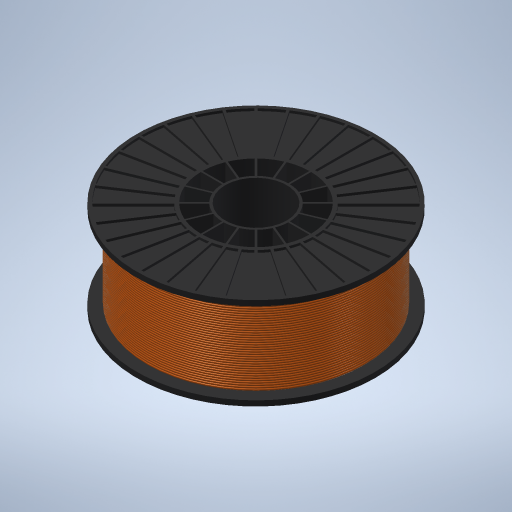
# Autodesk Inventor part: Sample Filament Spool
Saved by Autodesk Inventor 2024 (Build 280153000, 153)
## iProperties
Created: 2017-02-19
Part Number: Sample Filament Spool
Material: ABS Plastic
Document SubType Name: Modeling
Designer: Ishaan Govindarajan
Density: 1.06 g/cm^3
Appearance: Rubber - Black
Mass: 1663.72 g
Surface Area: 2295.81 cm^2
Volume: 1569.55 cm^3
Author: Ishaan Govindarajan
Autodesk Inventor part; units mm, degrees
ref_plane "YZ Plane" through (0, 0, 0) normal (1, 0, 0) x (0, 1, 0)
ref_plane "XZ Plane" through (0, 0, 0) normal (0, 1, 0) x (-1, 0, 0)
ref_plane "XY Plane" through (0, 0, 0) normal (0, 0, 1) x (1, 0, 0)
sketch "Sketch1" plane through (0, 0, 0) normal (0, 0, 1) x (1, 0, 0)
  circle A0 centre (0, 0) radius 101
  dimension "d0" = 202
  constraints: 1 centre point, 1 coincident
  measures "d0" diameter of A0
extrude "Extrusion1" add sketch "Sketch1" along normal mid plane 78
hole "Hole2" at (0, 0, 39) direction (0, 0, -1) diameter 52 end through all
sketch "Sketch4" plane through (0, 0, 39) normal (0, 0, 1) x (1, 0, 0)
  circle A0 centre (0, 0) radius 26 projected
  circle A1 centre (0, 0) radius 26 projected
  circle A2 centre (0, 0) radius 101 projected
  circle A3 centre (0, 0) radius 46
  circle A4 centre (0, 0) radius 28
  dimension "d22" = 20
  dimension "d23" = 2
  constraints: 2 centre point
  measures "d22" radial gap between concentric circles of A0 A3
  measures "d23" radial gap between concentric circles of A0 A4
extrude "Extrusion3" cut sketch "Sketch4" against normal blind 25 contours A3
sketch "Sketch5" plane through (0, 0, 39) normal (0, 0, 1) x (1, 0, 0)
  circle A0 centre (0, 0) radius 101 projected
  circle A1 centre (0, 0) radius 46 projected
  circle A2 centre (0, 0) radius 28 projected
  circle A3 centre (0, 0) radius 26 projected
  line L0 (-46, 0.75) -> (-27.99, 0.75)
  line L1 (-27.99, 0.75) -> (-27.99, -0.75)
  line L2 (-27.99, -0.75) -> (-46, -0.75)
  line L3 (-46, -0.75) -> (-46, 0.75)
  circle A4 centre (0, 0) radius 28 projected
  point P0 (-27.99, 0)
  dimension "d26" = 1.5
  constraints: 8 end point, 2 parallel, 1 horizontal, 1 horizontal alignment, 1 midpoint, 1 perpendicular, 1 tangent, 2 other
  measures "d26" distance of L2.end L0.start
extrude "Extrusion4" add sketch "Sketch5" against normal up to surface (25 mm away) contours L0 A2 L2 A1 | A1 L3 L0 | L2 L3 A1 | L1 A2 picked at (-33.9993, 0) picked at (-27.993, 0.0833)
pattern_circular "Circular Pattern1" count 16 over 360 about axis through (0, 0, -257.1284) along (0, 0, 1) of "Extrusion4"
sketch "Sketch6" plane through (0, 0, 39) normal (0, 0, 1) x (1, 0, 0)
  arc A0 (-33.0529, 31.9923) -> (-42.2058, 18.294) centre (0, 0) ccw projected
  line L0 (-20.3222, 19.2616) -> (-33.0529, 31.9923) projected
  arc A1 (-20.3222, 19.2616) -> (-25.5723, 11.4042) centre (0, 0) ccw projected
  line L1 (-42.2058, 18.294) -> (-25.5723, 11.4042) projected
  arc A2 (-18.294, 42.2058) -> (-31.9923, 33.0529) centre (0, 0) ccw projected
  line L2 (-11.4042, 25.5723) -> (-18.294, 42.2058) projected
  arc A3 (-11.4042, 25.5723) -> (-19.2616, 20.3222) centre (0, 0) ccw projected
  line L3 (-31.9923, 33.0529) -> (-19.2616, 20.3222) projected
  arc A4 (-0.75, 45.9939) -> (-16.9082, 42.7798) centre (0, 0) ccw projected
  line L4 (-0.75, 27.99) -> (-0.75, 45.9939) projected
  arc A5 (-0.75, 27.99) -> (-10.0184, 26.1464) centre (0, 0) ccw projected
  line L5 (-16.9082, 42.7798) -> (-10.0184, 26.1464) projected
  arc A6 (16.9082, 42.7798) -> (0.75, 45.9939) centre (0, 0) ccw projected
  line L6 (10.0184, 26.1464) -> (16.9082, 42.7798) projected
  arc A7 (10.0184, 26.1464) -> (0.75, 27.99) centre (0, 0) ccw projected
  line L7 (0.75, 45.9939) -> (0.75, 27.99) projected
  arc A8 (31.9923, 33.0529) -> (18.294, 42.2058) centre (0, 0) ccw projected
  line L8 (19.2616, 20.3222) -> (31.9923, 33.0529) projected
  arc A9 (19.2616, 20.3222) -> (11.4042, 25.5723) centre (0, 0) ccw projected
  line L9 (18.294, 42.2058) -> (11.4042, 25.5723) projected
  arc A10 (42.2058, 18.294) -> (33.0529, 31.9923) centre (0, 0) ccw projected
  line L10 (25.5723, 11.4042) -> (42.2058, 18.294) projected
  arc A11 (25.5723, 11.4042) -> (20.3222, 19.2616) centre (0, 0) ccw projected
  line L11 (33.0529, 31.9923) -> (20.3222, 19.2616) projected
  arc A12 (45.9939, 0.75) -> (42.7798, 16.9082) centre (0, 0) ccw projected
  line L12 (27.99, 0.75) -> (45.9939, 0.75) projected
  arc A13 (27.99, 0.75) -> (26.1464, 10.0184) centre (0, 0) ccw projected
  line L13 (42.7798, 16.9082) -> (26.1464, 10.0184) projected
  arc A14 (42.7798, -16.9082) -> (45.9939, -0.75) centre (0, 0) ccw projected
  line L14 (26.1464, -10.0184) -> (42.7798, -16.9082) projected
  arc A15 (26.1464, -10.0184) -> (27.99, -0.75) centre (0, 0) ccw projected
  line L15 (45.9939, -0.75) -> (27.99, -0.75) projected
  arc A16 (33.0529, -31.9923) -> (42.2058, -18.294) centre (0, 0) ccw projected
  line L16 (20.3222, -19.2616) -> (33.0529, -31.9923) projected
  arc A17 (20.3222, -19.2616) -> (25.5723, -11.4042) centre (0, 0) ccw projected
  line L17 (42.2058, -18.294) -> (25.5723, -11.4042) projected
  arc A18 (18.294, -42.2058) -> (31.9923, -33.0529) centre (0, 0) ccw projected
  line L18 (11.4042, -25.5723) -> (18.294, -42.2058) projected
  arc A19 (11.4042, -25.5723) -> (19.2616, -20.3222) centre (0, 0) ccw projected
  line L19 (31.9923, -33.0529) -> (19.2616, -20.3222) projected
  arc A20 (0.75, -45.9939) -> (16.9082, -42.7798) centre (0, 0) ccw projected
  line L20 (0.75, -27.99) -> (0.75, -45.9939) projected
  arc A21 (0.75, -27.99) -> (10.0184, -26.1464) centre (0, 0) ccw projected
  line L21 (16.9082, -42.7798) -> (10.0184, -26.1464) projected
  arc A22 (-16.9082, -42.7798) -> (-0.75, -45.9939) centre (0, 0) ccw projected
  line L22 (-10.0184, -26.1464) -> (-16.9082, -42.7798) projected
  arc A23 (-10.0184, -26.1464) -> (-0.75, -27.99) centre (0, 0) ccw projected
  line L23 (-0.75, -45.9939) -> (-0.75, -27.99) projected
  arc A24 (-31.9923, -33.0529) -> (-18.294, -42.2058) centre (0, 0) ccw projected
  line L24 (-19.2616, -20.3222) -> (-31.9923, -33.0529) projected
  arc A25 (-19.2616, -20.3222) -> (-11.4042, -25.5723) centre (0, 0) ccw projected
  line L25 (-18.294, -42.2058) -> (-11.4042, -25.5723) projected
  arc A26 (-42.2058, -18.294) -> (-33.0529, -31.9923) centre (0, 0) ccw projected
  line L26 (-25.5723, -11.4042) -> (-42.2058, -18.294) projected
  arc A27 (-25.5723, -11.4042) -> (-20.3222, -19.2616) centre (0, 0) ccw projected
  line L27 (-33.0529, -31.9923) -> (-20.3222, -19.2616) projected
  arc A28 (-45.9939, -0.75) -> (-42.7798, -16.9082) centre (0, 0) ccw projected
  line L28 (-27.99, -0.75) -> (-45.9939, -0.75) projected
  arc A29 (-27.99, -0.75) -> (-26.1464, -10.0184) centre (0, 0) ccw projected
  line L29 (-42.7798, -16.9082) -> (-26.1464, -10.0184) projected
  line L30 (-26.1464, 10.0184) -> (-42.7798, 16.9082) projected
  arc A30 (-26.1464, 10.0184) -> (-27.99, 0.75) centre (0, 0) ccw projected
  line L31 (-45.9939, 0.75) -> (-27.99, 0.75) projected
  arc A31 (-42.7798, 16.9082) -> (-45.9939, 0.75) centre (0, 0) ccw projected
  circle A32 centre (0, 0) radius 101 projected
  circle A33 centre (0, 0) radius 26 projected
  circle A34 centre (0, 0) radius 49
  circle A35 centre (0, 0) radius 98
  dimension "d32" = 3
  dimension "d33" = 3
  constraints: 2 centre point
  measures "d32" radial gap between concentric circles of A6 A34
  measures "d33" radial gap between concentric circles of A32 A35
extrude "Extrusion5" cut sketch "Sketch6" against normal blind 2 contours A35
sketch "Sketch7" plane through (0, 0, 37) normal (0, 0, 1) x (1, 0, 0)
  circle A0 centre (0, 0) radius 49 projected
  circle A1 centre (0, 0) radius 98 projected
  line L0 (-48.9898, 1) -> (-98, 1)
  line L1 (-98, 1) -> (-98, -1)
  line L2 (-98, -1) -> (-48.9898, -1)
  line L3 (-48.9898, -1) -> (-48.9898, 1)
  dimension "d36" = 2
  constraints: 8 end point, 2 parallel, 2 point on circle, 1 horizontal, 1 perpendicular, 1 tangent
  measures "d36" distance between parallel lines of L2 L0
extrude "Extrusion6" add sketch "Sketch7" along normal up to surface (2 mm away) contours A0 L2 A1 L0 | A1 L1 L0 | L2 L1 A1 picked at (-65.3326, 0)
pattern_circular "Circular Pattern2" count 32 over 360 about axis through (0, 0, 39) along (0, 0, -1) of "Extrusion6"
mirror "Mirror1" about plane through (0, 0, 0) normal (0, 0, 1) of "Extrusion3", "Extrusion4", "Circular Pattern1", "Extrusion5", "Extrusion6", "Circular Pattern2"
sketch "Sketch8" plane through (0, 0, -39) normal (0, 0, -1) x (-1, 0, 0)
  arc A0 (90.9182, -36.5771) -> (95.9169, -20.0986) centre (0, 0) ccw projected
  line L0 (90.9182, -36.5771) -> (45.6434, -17.8237) projected
  arc A1 (45.6434, -17.8237) -> (47.8534, -10.5382) centre (0, 0) ccw projected
  line L1 (47.8534, -10.5382) -> (95.9169, -20.0986) projected
  arc A2 (82.0353, -53.6116) -> (90.1528, -38.4249) centre (0, 0) ccw projected
  line L2 (82.0353, -53.6116) -> (41.2891, -26.3858) projected
  arc A3 (41.2891, -26.3858) -> (44.878, -19.6715) centre (0, 0) ccw projected
  line L3 (44.878, -19.6715) -> (90.1528, -38.4249) projected
  arc A4 (70, -68.5857) -> (80.9242, -55.2745) centre (0, 0) ccw projected
  line L4 (70, -68.5857) -> (35.3481, -33.9339) projected
  arc A5 (35.3481, -33.9339) -> (40.178, -28.0487) centre (0, 0) ccw projected
  line L5 (40.178, -28.0487) -> (80.9242, -55.2745) projected
  arc A6 (55.2745, -80.9242) -> (68.5857, -70) centre (0, 0) ccw projected
  line L6 (55.2745, -80.9242) -> (28.0487, -40.178) projected
  arc A7 (28.0487, -40.178) -> (33.9339, -35.3481) centre (0, 0) ccw projected
  line L7 (33.9339, -35.3481) -> (68.5857, -70) projected
  arc A8 (38.4249, -90.1528) -> (53.6116, -82.0353) centre (0, 0) ccw projected
  line L8 (38.4249, -90.1528) -> (19.6715, -44.878) projected
  arc A9 (19.6715, -44.878) -> (26.3858, -41.2891) centre (0, 0) ccw projected
  line L9 (26.3858, -41.2891) -> (53.6116, -82.0353) projected
  arc A10 (20.0986, -95.9169) -> (36.5771, -90.9182) centre (0, 0) ccw projected
  line L10 (20.0986, -95.9169) -> (10.5382, -47.8534) projected
  arc A11 (10.5382, -47.8534) -> (17.8237, -45.6434) centre (0, 0) ccw projected
  line L11 (17.8237, -45.6434) -> (36.5771, -90.9182) projected
  arc A12 (1, -97.9949) -> (18.1371, -96.307) centre (0, 0) ccw projected
  line L12 (1, -97.9949) -> (1, -48.9898) projected
  arc A13 (1, -48.9898) -> (8.5766, -48.2436) centre (0, 0) ccw projected
  line L13 (8.5766, -48.2436) -> (18.1371, -96.307) projected
  arc A14 (-18.1371, -96.307) -> (-1, -97.9949) centre (0, 0) ccw projected
  line L14 (-18.1371, -96.307) -> (-8.5766, -48.2436) projected
  arc A15 (-8.5766, -48.2436) -> (-1, -48.9898) centre (0, 0) ccw projected
  line L15 (-1, -48.9898) -> (-1, -97.9949) projected
  arc A16 (-36.5771, -90.9182) -> (-20.0986, -95.9169) centre (0, 0) ccw projected
  line L16 (-36.5771, -90.9182) -> (-17.8237, -45.6434) projected
  arc A17 (-17.8237, -45.6434) -> (-10.5382, -47.8534) centre (0, 0) ccw projected
  line L17 (-10.5382, -47.8534) -> (-20.0986, -95.9169) projected
  arc A18 (-53.6116, -82.0353) -> (-38.4249, -90.1528) centre (0, 0) ccw projected
  line L18 (-53.6116, -82.0353) -> (-26.3858, -41.2891) projected
  arc A19 (-26.3858, -41.2891) -> (-19.6715, -44.878) centre (0, 0) ccw projected
  line L19 (-19.6715, -44.878) -> (-38.4249, -90.1528) projected
  arc A20 (-68.5857, -70) -> (-55.2745, -80.9242) centre (0, 0) ccw projected
  line L20 (-68.5857, -70) -> (-33.9339, -35.3481) projected
  arc A21 (-33.9339, -35.3481) -> (-28.0487, -40.178) centre (0, 0) ccw projected
  line L21 (-28.0487, -40.178) -> (-55.2745, -80.9242) projected
  arc A22 (-80.9242, -55.2745) -> (-70, -68.5857) centre (0, 0) ccw projected
  line L22 (-80.9242, -55.2745) -> (-40.178, -28.0487) projected
  arc A23 (-40.178, -28.0487) -> (-35.3481, -33.9339) centre (0, 0) ccw projected
  line L23 (-35.3481, -33.9339) -> (-70, -68.5857) projected
  arc A24 (-90.1528, -38.4249) -> (-82.0353, -53.6116) centre (0, 0) ccw projected
  line L24 (-90.1528, -38.4249) -> (-44.878, -19.6715) projected
  arc A25 (-44.878, -19.6715) -> (-41.2891, -26.3858) centre (0, 0) ccw projected
  line L25 (-41.2891, -26.3858) -> (-82.0353, -53.6116) projected
  arc A26 (-95.9169, -20.0986) -> (-90.9182, -36.5771) centre (0, 0) ccw projected
  line L26 (-95.9169, -20.0986) -> (-47.8534, -10.5382) projected
  arc A27 (-47.8534, -10.5382) -> (-45.6434, -17.8237) centre (0, 0) ccw projected
  line L27 (-45.6434, -17.8237) -> (-90.9182, -36.5771) projected
  arc A28 (-97.9949, -1) -> (-96.307, -18.1371) centre (0, 0) ccw projected
  line L28 (-97.9949, -1) -> (-48.9898, -1) projected
  arc A29 (-48.9898, -1) -> (-48.2436, -8.5766) centre (0, 0) ccw projected
  line L29 (-48.2436, -8.5766) -> (-96.307, -18.1371) projected
  arc A30 (-96.307, 18.1371) -> (-97.9949, 1) centre (0, 0) ccw projected
  line L30 (-96.307, 18.1371) -> (-48.2436, 8.5766) projected
  arc A31 (-48.2436, 8.5766) -> (-48.9898, 1) centre (0, 0) ccw projected
  line L31 (-48.9898, 1) -> (-97.9949, 1) projected
  arc A32 (-90.9182, 36.5771) -> (-95.9169, 20.0986) centre (0, 0) ccw projected
  line L32 (-90.9182, 36.5771) -> (-45.6434, 17.8237) projected
  arc A33 (-45.6434, 17.8237) -> (-47.8534, 10.5382) centre (0, 0) ccw projected
  line L33 (-47.8534, 10.5382) -> (-95.9169, 20.0986) projected
  arc A34 (-82.0353, 53.6116) -> (-90.1528, 38.4249) centre (0, 0) ccw projected
  line L34 (-82.0353, 53.6116) -> (-41.2891, 26.3858) projected
  arc A35 (-41.2891, 26.3858) -> (-44.878, 19.6715) centre (0, 0) ccw projected
  line L35 (-44.878, 19.6715) -> (-90.1528, 38.4249) projected
  arc A36 (-70, 68.5857) -> (-80.9242, 55.2745) centre (0, 0) ccw projected
  line L36 (-70, 68.5857) -> (-35.3481, 33.9339) projected
  arc A37 (-35.3481, 33.9339) -> (-40.178, 28.0487) centre (0, 0) ccw projected
  line L37 (-40.178, 28.0487) -> (-80.9242, 55.2745) projected
  arc A38 (-55.2745, 80.9242) -> (-68.5857, 70) centre (0, 0) ccw projected
  line L38 (-55.2745, 80.9242) -> (-28.0487, 40.178) projected
  arc A39 (-28.0487, 40.178) -> (-33.9339, 35.3481) centre (0, 0) ccw projected
  line L39 (-33.9339, 35.3481) -> (-68.5857, 70) projected
  arc A40 (-38.4249, 90.1528) -> (-53.6116, 82.0353) centre (0, 0) ccw projected
  line L40 (-38.4249, 90.1528) -> (-19.6715, 44.878) projected
  arc A41 (-19.6715, 44.878) -> (-26.3858, 41.2891) centre (0, 0) ccw projected
  line L41 (-26.3858, 41.2891) -> (-53.6116, 82.0353) projected
  arc A42 (-20.0986, 95.9169) -> (-36.5771, 90.9182) centre (0, 0) ccw projected
  line L42 (-20.0986, 95.9169) -> (-10.5382, 47.8534) projected
  arc A43 (-10.5382, 47.8534) -> (-17.8237, 45.6434) centre (0, 0) ccw projected
  line L43 (-17.8237, 45.6434) -> (-36.5771, 90.9182) projected
  arc A44 (-1, 97.9949) -> (-18.1371, 96.307) centre (0, 0) ccw projected
  line L44 (-1, 97.9949) -> (-1, 48.9898) projected
  arc A45 (-1, 48.9898) -> (-8.5766, 48.2436) centre (0, 0) ccw projected
  line L45 (-8.5766, 48.2436) -> (-18.1371, 96.307) projected
  arc A46 (18.1371, 96.307) -> (1, 97.9949) centre (0, 0) ccw projected
  line L46 (18.1371, 96.307) -> (8.5766, 48.2436) projected
  arc A47 (8.5766, 48.2436) -> (1, 48.9898) centre (0, 0) ccw projected
  line L47 (1, 48.9898) -> (1, 97.9949) projected
  arc A48 (36.5771, 90.9182) -> (20.0986, 95.9169) centre (0, 0) ccw projected
  line L48 (36.5771, 90.9182) -> (17.8237, 45.6434) projected
  arc A49 (17.8237, 45.6434) -> (10.5382, 47.8534) centre (0, 0) ccw projected
  line L49 (10.5382, 47.8534) -> (20.0986, 95.9169) projected
  arc A50 (53.6116, 82.0353) -> (38.4249, 90.1528) centre (0, 0) ccw projected
  line L50 (53.6116, 82.0353) -> (26.3858, 41.2891) projected
  arc A51 (26.3858, 41.2891) -> (19.6715, 44.878) centre (0, 0) ccw projected
  line L51 (19.6715, 44.878) -> (38.4249, 90.1528) projected
  arc A52 (68.5857, 70) -> (55.2745, 80.9242) centre (0, 0) ccw projected
  line L52 (68.5857, 70) -> (33.9339, 35.3481) projected
  arc A53 (33.9339, 35.3481) -> (28.0487, 40.178) centre (0, 0) ccw projected
  line L53 (28.0487, 40.178) -> (55.2745, 80.9242) projected
  arc A54 (80.9242, 55.2745) -> (70, 68.5857) centre (0, 0) ccw projected
  line L54 (80.9242, 55.2745) -> (40.178, 28.0487) projected
  arc A55 (40.178, 28.0487) -> (35.3481, 33.9339) centre (0, 0) ccw projected
  line L55 (35.3481, 33.9339) -> (70, 68.5857) projected
  arc A56 (90.1528, 38.4249) -> (82.0353, 53.6116) centre (0, 0) ccw projected
  line L56 (90.1528, 38.4249) -> (44.878, 19.6715) projected
  arc A57 (44.878, 19.6715) -> (41.2891, 26.3858) centre (0, 0) ccw projected
  line L57 (41.2891, 26.3858) -> (82.0353, 53.6116) projected
  arc A58 (95.9169, 20.0986) -> (90.9182, 36.5771) centre (0, 0) ccw projected
  line L58 (95.9169, 20.0986) -> (47.8534, 10.5382) projected
  arc A59 (47.8534, 10.5382) -> (45.6434, 17.8237) centre (0, 0) ccw projected
  line L59 (45.6434, 17.8237) -> (90.9182, 36.5771) projected
  arc A60 (97.9949, 1) -> (96.307, 18.1371) centre (0, 0) ccw projected
  line L60 (97.9949, 1) -> (48.9898, 1) projected
  arc A61 (48.9898, 1) -> (48.2436, 8.5766) centre (0, 0) ccw projected
  line L61 (48.2436, 8.5766) -> (96.307, 18.1371) projected
  line L62 (42.7798, -16.9082) -> (26.1464, -10.0184) projected
  arc A62 (26.1464, -10.0184) -> (27.99, -0.75) centre (0, 0) ccw projected
  line L63 (27.99, -0.75) -> (45.9939, -0.75) projected
  arc A63 (42.7798, -16.9082) -> (45.9939, -0.75) centre (0, 0) ccw projected
  circle A64 centre (0, 0) radius 26 projected
  line L64 (33.0529, -31.9923) -> (20.3222, -19.2616) projected
  arc A65 (20.3222, -19.2616) -> (25.5723, -11.4042) centre (0, 0) ccw projected
  line L65 (25.5723, -11.4042) -> (42.2058, -18.294) projected
  arc A66 (33.0529, -31.9923) -> (42.2058, -18.294) centre (0, 0) ccw projected
  line L66 (18.294, -42.2058) -> (11.4042, -25.5723) projected
  arc A67 (11.4042, -25.5723) -> (19.2616, -20.3222) centre (0, 0) ccw projected
  line L67 (19.2616, -20.3222) -> (31.9923, -33.0529) projected
  arc A68 (18.294, -42.2058) -> (31.9923, -33.0529) centre (0, 0) ccw projected
  line L68 (0.75, -45.9939) -> (0.75, -27.99) projected
  arc A69 (0.75, -27.99) -> (10.0184, -26.1464) centre (0, 0) ccw projected
  line L69 (10.0184, -26.1464) -> (16.9082, -42.7798) projected
  arc A70 (0.75, -45.9939) -> (16.9082, -42.7798) centre (0, 0) ccw projected
  line L70 (-16.9082, -42.7798) -> (-10.0184, -26.1464) projected
  arc A71 (-10.0184, -26.1464) -> (-0.75, -27.99) centre (0, 0) ccw projected
  line L71 (-0.75, -27.99) -> (-0.75, -45.9939) projected
  arc A72 (-16.9082, -42.7798) -> (-0.75, -45.9939) centre (0, 0) ccw projected
  line L72 (-31.9923, -33.0529) -> (-19.2616, -20.3222) projected
  arc A73 (-19.2616, -20.3222) -> (-11.4042, -25.5723) centre (0, 0) ccw projected
  line L73 (-11.4042, -25.5723) -> (-18.294, -42.2058) projected
  arc A74 (-31.9923, -33.0529) -> (-18.294, -42.2058) centre (0, 0) ccw projected
  line L74 (-42.2058, -18.294) -> (-25.5723, -11.4042) projected
  arc A75 (-25.5723, -11.4042) -> (-20.3222, -19.2616) centre (0, 0) ccw projected
  line L75 (-20.3222, -19.2616) -> (-33.0529, -31.9923) projected
  arc A76 (-42.2058, -18.294) -> (-33.0529, -31.9923) centre (0, 0) ccw projected
  line L76 (-45.9939, -0.75) -> (-27.99, -0.75) projected
  arc A77 (-27.99, -0.75) -> (-26.1464, -10.0184) centre (0, 0) ccw projected
  line L77 (-26.1464, -10.0184) -> (-42.7798, -16.9082) projected
  arc A78 (-45.9939, -0.75) -> (-42.7798, -16.9082) centre (0, 0) ccw projected
  line L78 (-42.7798, 16.9082) -> (-26.1464, 10.0184) projected
  arc A79 (-26.1464, 10.0184) -> (-27.99, 0.75) centre (0, 0) ccw projected
  line L79 (-27.99, 0.75) -> (-45.9939, 0.75) projected
  arc A80 (-42.7798, 16.9082) -> (-45.9939, 0.75) centre (0, 0) ccw projected
  line L80 (-33.0529, 31.9923) -> (-20.3222, 19.2616) projected
  arc A81 (-20.3222, 19.2616) -> (-25.5723, 11.4042) centre (0, 0) ccw projected
  line L81 (-25.5723, 11.4042) -> (-42.2058, 18.294) projected
  arc A82 (-33.0529, 31.9923) -> (-42.2058, 18.294) centre (0, 0) ccw projected
  line L82 (-18.294, 42.2058) -> (-11.4042, 25.5723) projected
  arc A83 (-11.4042, 25.5723) -> (-19.2616, 20.3222) centre (0, 0) ccw projected
  line L83 (-19.2616, 20.3222) -> (-31.9923, 33.0529) projected
  arc A84 (-18.294, 42.2058) -> (-31.9923, 33.0529) centre (0, 0) ccw projected
  line L84 (-0.75, 45.9939) -> (-0.75, 27.99) projected
  arc A85 (-0.75, 27.99) -> (-10.0184, 26.1464) centre (0, 0) ccw projected
  line L85 (-10.0184, 26.1464) -> (-16.9082, 42.7798) projected
  arc A86 (-0.75, 45.9939) -> (-16.9082, 42.7798) centre (0, 0) ccw projected
  line L86 (16.9082, 42.7798) -> (10.0184, 26.1464) projected
  arc A87 (10.0184, 26.1464) -> (0.75, 27.99) centre (0, 0) ccw projected
  line L87 (0.75, 27.99) -> (0.75, 45.9939) projected
  arc A88 (16.9082, 42.7798) -> (0.75, 45.9939) centre (0, 0) ccw projected
  line L88 (31.9923, 33.0529) -> (19.2616, 20.3222) projected
  arc A89 (19.2616, 20.3222) -> (11.4042, 25.5723) centre (0, 0) ccw projected
  line L89 (11.4042, 25.5723) -> (18.294, 42.2058) projected
  arc A90 (31.9923, 33.0529) -> (18.294, 42.2058) centre (0, 0) ccw projected
  line L90 (42.2058, 18.294) -> (25.5723, 11.4042) projected
  arc A91 (25.5723, 11.4042) -> (20.3222, 19.2616) centre (0, 0) ccw projected
  line L91 (20.3222, 19.2616) -> (33.0529, 31.9923) projected
  arc A92 (42.2058, 18.294) -> (33.0529, 31.9923) centre (0, 0) ccw projected
  arc A93 (45.9939, 0.75) -> (42.7798, 16.9082) centre (0, 0) ccw projected
  line L92 (45.9939, 0.75) -> (27.99, 0.75) projected
  arc A94 (27.99, 0.75) -> (26.1464, 10.0184) centre (0, 0) ccw projected
  line L93 (26.1464, 10.0184) -> (42.7798, 16.9082) projected
  line L94 (96.307, -18.1371) -> (48.2436, -8.5766) projected
  arc A95 (48.2436, -8.5766) -> (48.9898, -1) centre (0, 0) ccw projected
  line L95 (48.9898, -1) -> (97.9949, -1) projected
  arc A96 (96.307, -18.1371) -> (97.9949, -1) centre (0, 0) ccw projected
  circle A97 centre (0, 0) radius 101 projected
  circle A98 centre (0, 0) radius 46
  constraints: 1 coincident, 3 other
extrude "Extrusion7" cut sketch "Sketch8" against normal blind 16 contours A98 L65 A65 L64 L67 A67 L66 L69 A69 L68 L71 A71 L70 L73 A73 L72 L75 A75 L74 L77 A77 L76 L79 A79 L78 L81 A81 L80 L83 A83 L82 L85 A85 L84 L87 A87 L86 L89 A89 L88 L91 A91 L90 L93 A94 L92 L63 A62 L62
sketch "Sketch9" plane through (42.2058, -18.294, -14) normal (0, 0, -1) x (-0.9238795, 0.3826834, 0)
  line L0 (14.0016, 33.8029) -> (26.7323, 21.0722) projected
  arc A0 (34.5897, 26.3223) -> (26.7323, 21.0722) centre (45.9939, 0.75) ccw projected
  line L1 (34.5897, 26.3223) -> (27.6999, 42.9558) projected
  arc A1 (27.6999, 42.9558) -> (14.0016, 33.8029) centre (45.9939, 0.75) ccw projected
  line L2 (29.0857, 43.5298) -> (35.9755, 26.8964) projected
  arc A2 (45.2439, 28.74) -> (35.9755, 26.8964) centre (45.9939, 0.75) ccw projected
  line L3 (45.2439, 28.74) -> (45.2439, 46.7439) projected
  arc A3 (45.2439, 46.7439) -> (29.0857, 43.5298) centre (45.9939, 0.75) ccw projected
  line L4 (46.7439, 46.7439) -> (46.7439, 28.74) projected
  arc A4 (56.0123, 26.8964) -> (46.7439, 28.74) centre (45.9939, 0.75) ccw projected
  line L5 (56.0123, 26.8964) -> (62.9021, 43.5298) projected
  arc A5 (62.9021, 43.5298) -> (46.7439, 46.7439) centre (45.9939, 0.75) ccw projected
  line L6 (64.2879, 42.9558) -> (57.3981, 26.3223) projected
  arc A6 (65.2554, 21.0722) -> (57.3981, 26.3223) centre (45.9939, 0.75) ccw projected
  line L7 (65.2554, 21.0722) -> (77.9861, 33.8029) projected
  arc A7 (77.9861, 33.8029) -> (64.2879, 42.9558) centre (45.9939, 0.75) ccw projected
  line L8 (79.0468, 32.7423) -> (66.3161, 20.0116) projected
  arc A8 (71.5662, 12.1542) -> (66.3161, 20.0116) centre (45.9939, 0.75) ccw projected
  line L9 (71.5662, 12.1542) -> (88.1997, 19.044) projected
  arc A9 (88.1997, 19.044) -> (79.0468, 32.7423) centre (45.9939, 0.75) ccw projected
  line L10 (88.7737, 17.6582) -> (72.1402, 10.7684) projected
  arc A10 (73.9838, 1.5) -> (72.1402, 10.7684) centre (45.9939, 0.75) ccw projected
  line L11 (73.9838, 1.5) -> (91.9878, 1.5) projected
  arc A11 (91.9878, 1.5) -> (88.7737, 17.6582) centre (45.9939, 0.75) ccw projected
  line L12 (91.9878, 0) -> (73.9838, 0) projected
  arc A12 (72.1402, -9.2684) -> (73.9838, 0) centre (45.9939, 0.75) ccw projected
  line L13 (72.1402, -9.2684) -> (88.7737, -16.1582) projected
  arc A13 (88.7737, -16.1582) -> (91.9878, 0) centre (45.9939, 0.75) ccw projected
  line L14 (88.1997, -17.544) -> (71.5662, -10.6542) projected
  arc A14 (66.3161, -18.5116) -> (71.5662, -10.6542) centre (45.9939, 0.75) ccw projected
  line L15 (66.3161, -18.5116) -> (79.0468, -31.2423) projected
  arc A15 (79.0468, -31.2423) -> (88.1997, -17.544) centre (45.9939, 0.75) ccw projected
  line L16 (3.7881, 19.044) -> (20.4216, 12.1542) projected
  arc A16 (25.6717, 20.0116) -> (20.4216, 12.1542) centre (45.9939, 0.75) ccw projected
  line L17 (25.6717, 20.0116) -> (12.941, 32.7423) projected
  arc A17 (12.941, 32.7423) -> (3.7881, 19.044) centre (45.9939, 0.75) ccw projected
  line L18 (0, 1.5) -> (18.0039, 1.5) projected
  arc A18 (19.8475, 10.7684) -> (18.0039, 1.5) centre (45.9939, 0.75) ccw projected
  line L19 (19.8475, 10.7684) -> (3.2141, 17.6582) projected
  arc A19 (3.2141, 17.6582) -> (0, 1.5) centre (45.9939, 0.75) ccw projected
  line L20 (3.2141, -16.1582) -> (19.8475, -9.2684) projected
  arc A20 (18.0039, 0) -> (19.8475, -9.2684) centre (45.9939, 0.75) ccw projected
  line L21 (18.0039, 0) -> (0, 0) projected
  arc A21 (0, 0) -> (3.2141, -16.1582) centre (45.9939, 0.75) ccw projected
  line L22 (12.941, -31.2423) -> (25.6717, -18.5116) projected
  arc A22 (20.4216, -10.6542) -> (25.6717, -18.5116) centre (45.9939, 0.75) ccw projected
  line L23 (20.4216, -10.6542) -> (3.7881, -17.544) projected
  arc A23 (3.7881, -17.544) -> (12.941, -31.2423) centre (45.9939, 0.75) ccw projected
  line L24 (27.6999, -41.4558) -> (34.5897, -24.8223) projected
  arc A24 (26.7323, -19.5722) -> (34.5897, -24.8223) centre (45.9939, 0.75) ccw projected
  line L25 (26.7323, -19.5722) -> (14.0016, -32.3029) projected
  arc A25 (14.0016, -32.3029) -> (27.6999, -41.4558) centre (45.9939, 0.75) ccw projected
  line L26 (45.2439, -45.2439) -> (45.2439, -27.24) projected
  arc A26 (35.9755, -25.3964) -> (45.2439, -27.24) centre (45.9939, 0.75) ccw projected
  line L27 (35.9755, -25.3964) -> (29.0857, -42.0298) projected
  arc A27 (29.0857, -42.0298) -> (45.2439, -45.2439) centre (45.9939, 0.75) ccw projected
  line L28 (57.3981, -24.8223) -> (64.2879, -41.4558) projected
  arc A28 (64.2879, -41.4558) -> (77.9861, -32.3029) centre (45.9939, 0.75) ccw projected
  line L29 (77.9861, -32.3029) -> (65.2554, -19.5722) projected
  arc A29 (57.3981, -24.8223) -> (65.2554, -19.5722) centre (45.9939, 0.75) ccw projected
  line L30 (62.9021, -42.0298) -> (56.0123, -25.3964) projected
  arc A30 (46.7439, -27.24) -> (56.0123, -25.3964) centre (45.9939, 0.75) ccw projected
  line L31 (46.7439, -27.24) -> (46.7439, -45.2439) projected
  arc A31 (46.7439, -45.2439) -> (62.9021, -42.0298) centre (45.9939, 0.75) ccw projected
  circle A32 centre (45.9939, 0.75) radius 26 projected
  circle A33 centre (45.9939, 0.75) radius 101 projected
extrude "Extrusion8" cut sketch "Sketch9" against normal blind 26 contours A1 L1 A0 L0 | A3 L3 A2 L2 | A5 L5 A4 L4 | A7 L7 A6 L6 | A9 L9 A8 L8 | A11 L11 A10 L10 | A13 L13 A12 L12 | A15 L15 A14 L14 | A17 L17 A16 L16 | A19 L19 A18 L18 | A21 L21 A20 L20 | A23 L23 A22 L22 | A25 L25 A24 L24 | A27 L27 A26 L26 | A29 L29 A28 L28 | A31 L31 A30 L30
sketch "Sketch10" plane through (0, 0, 0) normal (1, 0, 0) x (0, 1, 0)
  line L0 (-101, 39) -> (-26, 39) projected
  line L1 (-26, 39) -> (-26, -23) projected
  line L2 (-26, -23) -> (-46, -23) projected
  line L3 (-46, -23) -> (-46, -39) projected
  line L4 (-46, -39) -> (-101, -39) projected
  line L5 (-101, -39) -> (-101, 39) projected
  line L6 (26, 39) -> (101, 39) projected
  line L7 (101, 39) -> (101, -39) projected
  line L8 (101, -39) -> (46, -39) projected
  line L9 (46, -39) -> (46, -23) projected
  line L10 (46, -23) -> (26, -23) projected
  line L11 (26, -23) -> (26, 39) projected
  line L12 (101, -34.5) -> (91, -34.5)
  line L13 (91, -34.5) -> (91, 34.5)
  line L14 (91, 34.5) -> (101, 34.5)
  line L15 (101, 34.5) -> (101, -34.5)
  line L16 (0, -54.6) -> (0, 54.6) projected
  point P0 (0, 0)
  dimension "d46" = 4.5
  dimension "d47" = 4.5
  dimension "d48" = 10
  constraints: 8 end point, 2 parallel, 1 horizontal, 1 perpendicular, 1 point on line
  measures "d46" distance between parallel lines of L12 L8
  measures "d47" distance between parallel lines of L6 L14
  measures "d48" distance between parallel lines of L7 L13
revolve "Revolution1" cut sketch "Sketch10" angle 360 about axis through (0, 0, -10) along (0, 0, 1) contours L7 L12 L13 L14
sketch "Sketch11" plane through (0, 0, 0) normal (1, 0, 0) x (0, 1, 0)
  line L0 (91, -34.5) -> (-91, -34.5) projected
  line L1 (91, 34.5) -> (-91, 34.5) projected
  line L2 (-101, 39) -> (-26, 39) projected
  line L3 (-26, 39) -> (-26, -23) projected
  line L4 (-26, -23) -> (-46, -23) projected
  line L5 (-46, -23) -> (-46, -39) projected
  line L6 (-46, -39) -> (-101, -39) projected
  line L7 (-101, -39) -> (-101, -34.5) projected
  line L8 (-101, -34.5) -> (-91, -34.5) projected
  line L9 (-91, -34.5) -> (-91, 34.5) projected
  line L10 (-91, 34.5) -> (-101, 34.5) projected
  line L11 (-101, 34.5) -> (-101, 39) projected
  line L12 (26, 39) -> (101, 39) projected
  line L13 (101, 39) -> (101, 34.5) projected
  line L14 (101, 34.5) -> (91, 34.5) projected
  line L15 (91, 34.5) -> (91, -34.5) projected
  line L16 (91, -34.5) -> (101, -34.5) projected
  line L17 (101, -34.5) -> (101, -39) projected
  line L18 (101, -39) -> (46, -39) projected
  line L19 (46, -39) -> (46, -23) projected
  line L20 (46, -23) -> (26, -23) projected
  line L21 (26, -23) -> (26, 39) projected
  circle A0 centre (91, -33.625) radius 0.875
  line L22 (0, -54.6) -> (0, 54.6) projected
  point P0 (0, 0)
  dimension "d50" = 69
  dimension "d51" = 1.75
  constraints: 1 centre point, 1 point on line, 1 tangent
  measures "d50" distance of L1.start L0.start
  measures "d51" diameter of A0
revolve "Revolution2" add sketch "Sketch11" angle 360 about axis through (0, 0, -10) along (0, 0, 1) contours A0 L15 | L15 A0
pattern_linear "Rectangular Pattern1" count 40 spacing 1.75 along (0, 0, 1) of "Revolution2"
body "Solid1"
